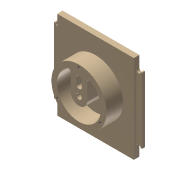
# Autodesk Inventor part: JointB0
Saved by Autodesk Inventor 2013 (Build 170138000, 138)
## iProperties
Created: 2012-10-15
Part Number: JointB0
Document SubType Name: Modeling
Designer: JohnHenry
Density: 0.952 g/cm^3
Material: ポリエチレン、低密度
Mass: 42.3609 g
Surface Area: 197.869 cm^2
Volume: 44.4968 cm^3
Author: JohnHenry
Autodesk Inventor part; units mm, degrees
ref_plane "YZ Plane" through (0, 0, 0) normal (1, 0, 0) x (0, 1, 0)
ref_plane "XZ Plane" through (0, 0, 0) normal (0, 1, 0) x (-1, 0, 0)
ref_plane "XY Plane" through (0, 0, 0) normal (0, 0, 1) x (1, 0, 0)
sketch "スケッチ1" plane through (0, 0, 0) normal (0, 0, 1) x (1, 0, 0)
  line L0 (-40, 5) -> (40, 5)
  line L1 (40, 5) -> (40, 0)
  line L2 (40, 0) -> (-40, 0)
  line L3 (-40, 0) -> (-40, 5)
  point P0 (0, 0)
  dimension "d5" = 40
  dimension "d6" = 80
  dimension "d7" = 5
  dimension "d8" = 0
  constraints: 8 end point, 2 parallel, 1 horizontal, 1 perpendicular
  measures "d5" distance from line of L1 point (0, 0)
  measures "d6" distance of L0.start L0.end
  measures "d7" distance of L0.end L1.end
  measures "d8" distance from line of point (0, 0) L2
extrude "押し出し1" add sketch "スケッチ1" along normal blind 80
sketch "スケッチ5" plane through (-40, 0, 0) normal (0, -1, 0) x (1, 0, 0)
  circle A0 centre (40, 40) radius 25
  point P0 (40, 0)
  dimension "d19" = 50
  constraints: 1 centre point
  measures "d19" diameter of A0
extrude "押し出し4" add sketch "スケッチ5" along normal blind 15
sketch "スケッチ6" plane through (0, -15, 40) normal (0, -1, 0) x (1, 0, 0)
  circle A0 centre (0, 0) radius 25 projected
  circle A1 centre (0, 0) radius 2.5
  point P0 (0, -40)
  dimension "d22" = 5
  constraints: 1 centre point, 1 coincident
  measures "d22" diameter of A1
extrude "押し出し5" cut sketch "スケッチ6" against normal blind 20 contours A1
sketch "スケッチ10" plane through (-40, 0, 0) normal (0, -1, 0) x (1, 0, 0)
  line L0 (80, 0) -> (0, 0) projected
  line L1 (80, 0) -> (80, 80) projected
  line L2 (0, 80) -> (5.2, 80)
  line L3 (5.2, 80) -> (5.2, 0)
  line L4 (5.2, 0) -> (0, 0)
  line L5 (0, 0) -> (0, 80)
  line L6 (80, 80) -> (74.8, 80)
  line L7 (74.8, 80) -> (74.8, 0)
  line L8 (74.8, 0) -> (80, 0)
  line L9 (80, 0) -> (80, 80)
  point P0 (40, 0)
  dimension "d70" = 5.2
  dimension "d71" = 5.2
  constraints: 16 end point, 4 parallel, 2 horizontal, 2 perpendicular, 2 point on line
  measures "d70" distance between parallel lines of L5 L3
  measures "d71" distance between parallel lines of L1 L7
extrude "押し出し9" cut sketch "スケッチ10" against normal blind 2.2
sketch "スケッチ11" plane through (-40, 2.2, 0) normal (0, -1, 0) x (1, 0, 0)
  line L0 (5.2, 0) -> (5.2, 80) projected
  line L1 (0, 80) -> (5.2, 80)
  line L2 (5.2, 80) -> (5.2, 69.9)
  line L3 (5.2, 69.9) -> (0, 69.9)
  line L4 (0, 69.9) -> (0, 80)
  line L5 (0, 0) -> (5.2, 0)
  line L6 (5.2, 0) -> (5.2, 10.1)
  line L7 (5.2, 10.1) -> (0, 10.1)
  line L8 (0, 10.1) -> (0, 0)
  point P0 (40, 0)
  dimension "d76" = 10.1
  dimension "d77" = 10.1
  constraints: 16 end point, 4 parallel, 2 horizontal, 2 perpendicular, 2 point on line
  measures "d76" distance of L1.end L2.end
  measures "d77" distance of L5.end L6.end
extrude "押し出し10" cut sketch "スケッチ11" against normal through all
sketch "スケッチ12" plane through (-40, 2.2, 0) normal (0, -1, 0) x (1, 0, 0)
  line L0 (74.8, 80) -> (74.8, 0) projected
  line L1 (74.8, 80) -> (80, 80) projected
  line L2 (80, 80) -> (74.8, 80)
  line L3 (74.8, 80) -> (74.8, 69.9)
  line L4 (74.8, 69.9) -> (80, 69.9)
  line L5 (80, 69.9) -> (80, 80)
  line L6 (80, 0) -> (74.8, 0)
  line L7 (74.8, 0) -> (74.8, 10.1)
  line L8 (74.8, 10.1) -> (80, 10.1)
  line L9 (80, 10.1) -> (80, 0)
  point P0 (40, 0)
  dimension "d80" = 10.1
  dimension "d81" = 10.1
  constraints: 16 end point, 4 parallel, 2 horizontal, 2 perpendicular, 2 point on line
  measures "d80" distance of L6.end L7.end
  measures "d81" distance between parallel lines of L1 L4
extrude "押し出し11" cut sketch "スケッチ12" against normal through all
sketch "スケッチ13" plane through (-34.8, 5, 0) normal (0, 1, 0) x (1, 0, 0)
  line L0 (74.8, -10.1) -> (69.6, -10.1) projected
  line L1 (0, 0) -> (0, -10.1) projected
  line L2 (0, -10.1) -> (-5.2, -10.1) projected
  line L3 (-5.2, -69.9) -> (0, -69.9) projected
  line L4 (69.6, -80) -> (69.6, -69.9) projected
  line L5 (69.6, -69.9) -> (74.8, -69.9) projected
  point P0 (34.8, 0)
  point P1 (-2, -10.1)
  point P2 (-2, -69.9)
  point P3 (71.6, -69.9)
  point P4 (71.6, -10.1)
  dimension "d84" = 2
  dimension "d85" = 2
  dimension "d86" = 2
  dimension "d87" = 2
  constraints: 4 point on line
  measures "d84" distance from line of L1 point (-2, -10.1)
  measures "d85" distance of L3.end point (-2, -69.9)
  measures "d86" distance of L0.end point (71.6, -10.1)
  measures "d87" distance from line of L4 point (71.6, -69.9)
hole "Hole2" at (-36.8, 5, 10.1) at (-36.8, 5, 69.9) at (36.8, 5, 69.9) at (36.8, 5, 10.1) direction (0, -1, 0) diameter 4 end through all
sketch "スケッチ14" plane through (0, -15, 40) normal (0, -1, 0) x (1, 0, 0)
  circle A0 centre (0, 0) radius 2.5 projected
  line L0 (-2.5, 16) -> (2.5, 16)
  line L1 (2.5, 16) -> (2.5, 6)
  line L2 (2.5, 6) -> (-2.5, 6)
  line L3 (-2.5, 6) -> (-2.5, 16)
  point P0 (0, -40)
  dimension "d95" = 5
  dimension "d96" = 6
  dimension "d97" = 10
  constraints: 8 end point, 2 parallel, 1 horizontal, 1 perpendicular
  measures "d95" distance of L0.start L0.end
  measures "d96" distance from line of A0.centre L2
  measures "d97" distance of L0.end L1.end
extrude "押し出し12" cut sketch "スケッチ14" against normal through all contours L0 L1 L2 L3
fillet "フィレット6" radius 2 4 edges at (-2.5, -5, 56) (2.5, -5, 56) (2.5, -5, 46) (-2.5, -5, 46)
sketch "スケッチ16" plane through (0, -15, 40) normal (0, -1, 0) x (1, 0, 0)
  line L0 (-2.5, 8) -> (-2.5, 14) projected
  line L1 (2.5, 14) -> (2.5, 8) projected
  line L2 (0.5, 6) -> (-0.5, 6) projected
  circle A0 centre (0, 0) radius 2.5 projected
  circle A1 centre (0, 0) radius 25 projected
  arc A2 (-7.5, 18.5405) -> (7.5, 18.5405) centre (0, 0) ccw
  line L3 (-7.5, 18.5405) -> (-7.5, -7.5)
  line L4 (-7.5, -7.5) -> (7.5, -7.5)
  line L5 (7.5, -7.5) -> (7.5, 18.5405)
  arc A3 (7.5, 18.5405) -> (-7.5, 18.5405) centre (0, 0) ccw
  point P0 (0, -40)
  dimension "d104" = 40
  dimension "d105" = 5
  dimension "d106" = 5
  dimension "d107" = 7.5
  constraints: 6 end point, 4 point on circle, 2 centre point, 2 perpendicular, 1 coincident, 1 parallel
  measures "d104" diameter of A2
  measures "d105" distance between parallel lines of L3 L0
  measures "d106" distance between parallel lines of L1 L5
  measures "d107" distance from line of L4 A0.centre
extrude "押し出し14" cut sketch "スケッチ16" against normal up to surface (15 mm away) contours L3 L4 L5 A2
fillet "フィレット7" radius 7.5 2 edges at (7.5, -7.5, 32.5) (-7.5, -7.5, 32.5)
fillet "フィレット8" radius 2 2 edges at (7.5, -7.5, 58.5405) (-7.5, -7.5, 58.5405)
sketch "スケッチ17" plane through (0, -15, 40) normal (0, -1, 0) x (1, 0, 0)
  line L0 (0.5, 6) -> (-0.5, 6) projected
  circle A0 centre (0, 0) radius 2.5 projected
  circle A1 centre (0, 0) radius 22.5
  line L1 (0, 0) -> (0, 22.5)
  line L2 (0, 0) -> (19.4856, -11.25)
  line L3 (0, 0) -> (-19.4856, -11.25)
  point P0 (0, -40)
  point P1 (19.4856, -11.25)
  dimension "d112" = 45
  dimension "d113" = 120
  dimension "d114" = 120
  constraints: 6 end point, 4 point on circle, 3 coincident, 1 centre point, 1 perpendicular
  measures "d112" diameter of A1
  measures "d113" angle of L2 L1
  measures "d114" angle of L3 L2
hole "Hole3" at (0, -15, 62.5) at (19.4856, -15, 28.75) at (-19.4856, -15, 28.75) direction (0, 1, 0) diameter 2.459 end through all thread size "M3x0.5" class "6H" standard "ISO Metric profile"
equation "\"d5\" = 0.5 * d6"
equation "\"d9\" = d6"
equation "\"d77\" = d76"
equation "\"d81\" = d80"
equation "\"d85\" = d84"
equation "\"d86\" = d84"
equation "\"d87\" = d84"
